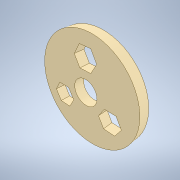
# Autodesk Inventor part: Бортик внутренний (конусной катушки)
Saved by Autodesk Inventor 2021.1 (Build 251245010, 245A)
## iProperties
Created: 2026-04-13
Part Number: Бортик внутренний (конусной катушки)
Material: Типовые
Document SubType Name: Modeling
Designer: Андрей Тарасов
Density: 1 g/cm^3
Appearance: По умолчанию
Author: Андрей Тарасов
Autodesk Inventor part; units mm, degrees
ref_plane "YZ Plane" through (0, 0, 0) normal (1, 0, 0) x (0, 1, 0)
ref_plane "XZ Plane" through (0, 0, 0) normal (0, 1, 0) x (-1, 0, 0)
ref_plane "XY Plane" through (0, 0, 0) normal (0, 0, 1) x (1, 0, 0)
sketch "Эскиз1" plane through (0, 0, 0) normal (0, 0, 1) x (1, 0, 0)
  circle A0 centre (0, 0) radius 5
  circle A1 centre (0, 0) radius 20.7
  line L0 (0, -28.98) -> (0, 28.98) construction
  line L1 (-28.98, 0) -> (28.98, 0) construction
  line L2 (2.3094, 8) -> (-2.3094, 8)
  line L3 (-2.3094, 8) -> (-4.6188, 12)
  line L4 (-4.6188, 12) -> (-2.3094, 16)
  line L5 (-2.3094, 16) -> (2.3094, 16)
  line L6 (2.3094, 16) -> (4.6188, 12)
  line L7 (4.6188, 12) -> (2.3094, 8)
  line L8 (-8.0829, -10) -> (-12.7017, -10)
  line L9 (-5.7735, -6) -> (-8.0829, -10)
  line L10 (-8.0829, -2) -> (-5.7735, -6)
  line L11 (-12.7017, -2) -> (-8.0829, -2)
  line L12 (-15.0111, -6) -> (-12.7017, -2)
  line L13 (-12.7017, -10) -> (-15.0111, -6)
  line L14 (12.7017, -2) -> (15.0111, -6)
  line L15 (8.0829, -2) -> (12.7017, -2)
  line L16 (5.7735, -6) -> (8.0829, -2)
  line L17 (8.0829, -10) -> (5.7735, -6)
  line L18 (12.7017, -10) -> (8.0829, -10)
  line L19 (15.0111, -6) -> (12.7017, -10)
  point P0 (0, 12)
  dimension "d0" = 10
  dimension "d1" = 41.4
  dimension "d10" = 12
  dimension "d11" = 8
  dimension "d14" = 360
  constraints: 36 end point, 2 centre point, 2 coincident, 1 horizontal, 1 point on line, 50 other
  measures "d0" diameter of A0
  measures "d1" diameter of A1
  measures "d10" distance of point (0, 12) point (0, 0)
  measures "d11" distance between parallel lines of L2 L5
extrude "Выдавливание1" add sketch "Эскиз1" along normal blind 4
